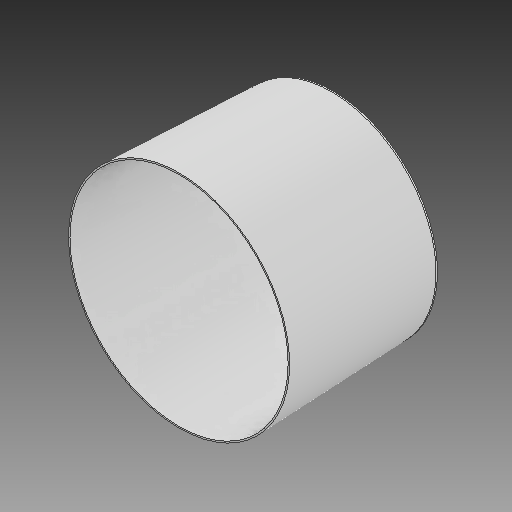
# Autodesk Inventor part: Abdeckungsrohr
Saved by Autodesk Inventor 2021 (Build 250183000, 183)
## iProperties
Created: 2022-02-23
Part Number: Abdeckungsrohr
Material: Generisch
Document SubType Name: Modeling
Designer: lukas
Density: 1 g/cm^3
Appearance: Vorgabe
Stock Number: Schutzrohr
Author: lukas
Autodesk Inventor part; units mm, degrees
ref_plane "YZ Plane" through (0, 0, 0) normal (1, 0, 0) x (0, 1, 0)
ref_plane "XZ Plane" through (0, 0, 0) normal (0, 1, 0) x (-1, 0, 0)
ref_plane "XY Plane" through (0, 0, 0) normal (0, 0, 1) x (1, 0, 0)
sketch "Skizze3" plane through (0, 0, 0) normal (0, 0, 1) x (1, 0, 0)
  line L0 (-201.6, 0) -> (201.6, 0) projected
  line L1 (0, -201.6) -> (0, 201.6) projected
  circle A0 centre (0, 0) radius 144
  dimension "d4" = 288
  constraints: 1 centre point, 1 coincident
  measures "d4" diameter of A0
extrude "Extrusion2" add sketch "Skizze3" along normal blind 210 draft 2.25
sketch "Skizze4" plane through (0, 0, 210) normal (0, 0, 1) x (1, 0, 0)
  circle A0 centre (0, 0) radius 150.2509
  circle A1 centre (0, 0) radius 152.2509 projected
  dimension "d7" = 2
  constraints: 1 centre point, 1 coincident
  measures "d7" radial gap between concentric circles of A1 A0
extrude "Extrusion3" cut sketch "Skizze4" against normal blind 210 draft -2.25 contours A0
sketch "Skizze5" plane through (0, 0, 0) normal (0, 0, -1) x (-1, 0, 0)
  circle A0 centre (0, 0) radius 144 projected
  circle A1 centre (0, 0) radius 144
  circle A2 centre (0, 0) radius 142
  constraints: 2 centre point, 2 coincident
extrude "Extrusion4" add sketch "Skizze5" along normal blind 2
